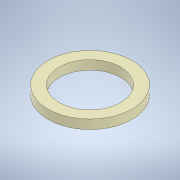
# Autodesk Inventor part: Skive_stempel_stang
Saved by Autodesk Inventor 2022 (Build 260153000, 153)
## iProperties
Created: 2022-04-10
Part Number: Skive_stempel_stang
Material: Polypropylene
Document SubType Name: Modeling
Designer: Patrick
Density: 0.899 g/cm^3
Appearance: Smooth - Ash
Mass: 0.553065 g
Surface Area: 8.22987 cm^2
Volume: 0.6152 cm^3
Author: Patrick
Autodesk Inventor part; units mm, degrees
ref_plane "YZ Plane" through (0, 0, 0) normal (1, 0, 0) x (0, 1, 0)
ref_plane "XZ Plane" through (0, 0, 0) normal (0, 1, 0) x (-1, 0, 0)
ref_plane "XY Plane" through (0, 0, 0) normal (0, 0, 1) x (1, 0, 0)
sketch "Sketch1" plane through (0, 0, 0) normal (0, 1, 0) x (-1, 0, 0)
  circle A0 centre (0, 0) radius 9.15
  circle A1 centre (0, 0) radius 12.5
  dimension "d0" = 18.3
  dimension "d1" = 25
  constraints: 2 centre point, 2 coincident
  measures "d0" diameter of A0
  measures "d1" diameter of A1
extrude "Extrusion1" add sketch "Sketch1" along normal blind 2.7
body "Solid1"
